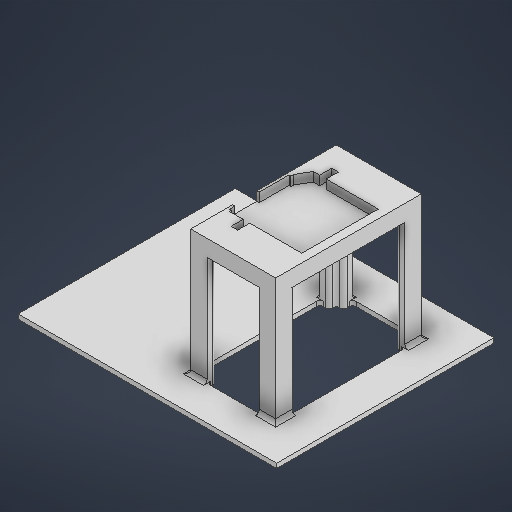
# Autodesk Inventor part: OMG_20kg_servo_side_profile(0.4mm)
Saved by Autodesk Inventor 2026.1 (Build 301233020, 233B)
## iProperties
Created: 2026-02-21
Part Number: OMG_20kg_servo_side_profile(0.4mm)
Material: Generic
Document SubType Name: Modeling
Designer: Lars
Density: 1 g/cm^3
Appearance: Default
Author: Lars
Autodesk Inventor part; units mm, degrees
ref_plane "YZ Plane" through (0, 0, 0) normal (1, 0, 0) x (0, 1, 0)
ref_plane "XZ Plane" through (0, 0, 0) normal (0, 1, 0) x (-1, 0, 0)
ref_plane "XY Plane" through (0, 0, 0) normal (0, 0, 1) x (1, 0, 0)
sketch "Sketch1" plane through (0, 0, 0) normal (0, 1, 0) x (-1, 0, 0)
  line L0 (0, 0) -> (28.63, 0)
  line L1 (28.63, 0) -> (28.63, -41.25) construction
  line L2 (28.63, -41.25) -> (0, -41.25)
  line L3 (0, -41.25) -> (0, 0)
  line L4 (28.63, 6.675) -> (31.43, 6.675)
  line L5 (31.43, 6.675) -> (31.43, 0)
  line L6 (31.43, -47.925) -> (28.63, -47.925)
  line L7 (28.63, -47.925) -> (28.63, -41.25)
  line L8 (31.43, -20.625) -> (28.63, -20.625) construction
  line L9 (38.98, 0) -> (31.43, 0)
  line L10 (31.43, 0) -> (31.43, -41.25) construction
  line L11 (31.43, -41.25) -> (35.18, -41.25)
  line L12 (38.98, -41.25) -> (38.98, -34.5) construction
  line L13 (31.43, -41.25) -> (35.18, -41.25) construction
  line L14 (38.98, 0) -> (38.98, -1) construction
  line L15 (38.98, -34.5) -> (35.18, -41.25)
  line L16 (38.98, -34.5) -> (38.98, -33)
  line L17 (35.18, -41.25) -> (38.98, -41.25) construction
  line L18 (38.98, 0) -> (38.98, -1) construction
  line L19 (38.98, -1) -> (39.98, -1)
  line L20 (39.98, -1) -> (39.98, -4)
  line L21 (39.98, -33) -> (38.98, -33)
  line L22 (38.98, -33) -> (38.98, -1) construction
  line L23 (38.98, -1) -> (38.98, -33) construction
  line L24 (38.98, -33) -> (38.98, -34.5) construction
  line L25 (38.98, -1) -> (38.98, 0)
  line L26 (38.98, -33) -> (38.98, -1) construction
  line L27 (31.43, 0) -> (31.43, -41.25) construction
  line L28 (31.43, -41.25) -> (31.43, -47.925)
  line L29 (28.63, -41.25) -> (28.63, 0) construction
  line L30 (28.63, 0) -> (28.63, 6.675)
  line L31 (28.63, 0) -> (31.43, 0) construction
  line L32 (31.43, -41.25) -> (28.63, -41.25) construction
  line L33 (39.98, -1) -> (39.98, -4) construction
  line L34 (39.98, -4) -> (41.28, -4)
  line L35 (41.28, -4) -> (41.28, -16.6)
  line L36 (41.28, -16.6) -> (39.98, -16.6)
  line L37 (39.98, -16.6) -> (39.98, -4) construction
  line L38 (39.98, -4) -> (39.98, -16.6) construction
  line L39 (39.98, -16.6) -> (39.98, -33)
  line L40 (41.68, -17) -> (41.68, -3.6)
  line L41 (41.68, -3.6) -> (40.38, -3.6)
  line L42 (40.38, -3.6) -> (40.38, -0.6)
  line L43 (40.38, -0.6) -> (39.38, -0.6)
  line L44 (39.38, -0.6) -> (39.38, 0.4)
  line L45 (39.38, 0.4) -> (31.83, 0.4)
  line L46 (31.83, 0.4) -> (31.83, 7.075)
  line L47 (31.83, 7.075) -> (28.23, 7.075)
  line L48 (28.23, 7.075) -> (28.23, 0.4)
  line L49 (28.23, 0.4) -> (-0.4, 0.4)
  line L50 (-0.4, 0.4) -> (-0.4, -41.65)
  line L51 (-0.4, -41.65) -> (28.23, -41.65)
  line L52 (28.23, -41.65) -> (28.23, -48.325)
  line L53 (28.23, -48.325) -> (31.83, -48.325)
  line L54 (31.83, -48.325) -> (31.83, -41.65)
  line L55 (31.83, -41.65) -> (35.4138, -41.65)
  line L56 (35.4138, -41.65) -> (39.38, -34.6049)
  line L57 (39.38, -34.6049) -> (39.38, -33.4)
  line L58 (39.38, -33.4) -> (40.38, -33.4)
  line L59 (40.38, -33.4) -> (40.38, -17)
  line L60 (40.38, -17) -> (41.68, -17)
  line L61 (0, -20.625) -> (39.98, -20.625) construction
  line L62 (44.99, 9.375) -> (-5.01, 9.375)
  line L63 (-5.01, 9.375) -> (-5.01, -50.625)
  line L64 (-5.01, -50.625) -> (44.99, -50.625)
  line L65 (44.99, -50.625) -> (44.99, 9.375)
  line L66 (19.99, 9.375) -> (19.99, -50.625) construction
  point P0 (30.03, 6.675)
  point P1 (19.99, -20.625)
  dimension "d0" = 28.63
  dimension "d1" = 41.25
  dimension "d2" = 2.8
  dimension "d3" = 54.6
  dimension "d4" = 7.55
  dimension "d5" = 41.25
  dimension "d6" = 3.75
  dimension "d7" = 34.5
  dimension "d8" = 1
  dimension "d9" = 32
  dimension "d10" = 1
  dimension "d11" = 6.675
  dimension "d12" = 3
  dimension "d13" = 1.3
  dimension "d14" = 12.6
  dimension "d15" = 0.4
  dimension "d16" = 50
  dimension "d17" = 60
  constraints: 134 end point, 35 parallel, 17 perpendicular, 8 midpoint, 7 horizontal, 5 vertical, 1 point on line, 20 other
  measures "d0" distance of L1.end L2.end
  measures "d1" distance of L0.end L1.end
  measures "d2" distance of L6.start L6.end
  measures "d3" distance of L4.end L6.start
  measures "d4" distance of L12.start L10.end
  measures "d5" distance of L12.start L9.start
  measures "d6" distance of L10.end L11.end
  measures "d7" distance of L9.start L12.end
  measures "d8" distance of L9.start L14.end
  measures "d9" distance of L19.end L21.start
  measures "d10" distance of L21.start L16.end
  measures "d11" distance from line of point (30.03, 6.675) L31
  measures "d12" distance of L19.end L20.end
  measures "d13" distance of L35.end L36.end
  measures "d14" distance of L34.end L35.end
  measures "d15" distance between parallel lines of L35 L40
  measures "d16" distance of L64.end L63.end
  measures "d17" distance of L63.end L62.end
extrude "Extrusion1" add sketch "Sketch1" along normal blind 5 contours L65 L64 L63 L62
sketch "Sketch2" plane through (0, 5, 0) normal (0, 1, 0) x (1, 0, 0)
  line L0 (-44.99, 50.625) -> (-44.99, -9.375) projected
  line L1 (5.01, 50.625) -> (-44.99, 50.625) projected
  line L2 (-44.99, -9.375) -> (-41.68, -9.375)
  line L3 (-41.68, -9.375) -> (-41.68, 50.625)
  line L4 (-41.68, 50.625) -> (-44.99, 50.625)
  line L5 (-44.99, 50.625) -> (-44.99, -9.375)
  point P0 (0, 0)
  dimension "d20" = 3.31
  constraints: 8 end point, 2 parallel, 1 horizontal, 1 perpendicular, 1 point on line
  measures "d20" distance of L4.end L3.end
extrude "Extrusion2" cut sketch "Sketch2" against normal through all
sketch "Sketch3" plane through (0, 0, 0) normal (0, -1, 0) x (1, 0, 0)
  line L0 (5.01, 9.375) -> (5.01, -50.625) projected
  line L1 (-41.68, -17) -> (-41.68, -50.625) projected
  line L2 (5.01, 9.375) -> (-41.68, 9.375)
  line L3 (-41.68, 9.375) -> (-41.68, -50.625)
  line L4 (-41.68, -50.625) -> (5.01, -50.625)
  line L5 (5.01, -50.625) -> (5.01, 9.375)
  point P0 (0, 0)
  constraints: 8 end point, 2 parallel, 1 horizontal, 1 perpendicular
extrude "Extrusion3" add sketch "Sketch3" along normal blind 4
sketch "Sketch4" plane through (-41.68, 5, 9.375) normal (0, 0, 1) x (1, 0, 0)
  line L0 (0, 0) -> (0, -9) projected
  line L1 (46.69, -9) -> (46.69, 0) projected
  line L2 (0, 0) -> (46.69, 0)
  line L3 (46.69, 0) -> (46.69, -9)
  line L4 (46.69, -9) -> (0, -9)
  line L5 (0, -9) -> (0, 0)
  point P0 (41.68, -5)
  constraints: 8 end point, 2 parallel, 1 horizontal, 1 perpendicular
extrude "Extrusion4" add sketch "Sketch4" along normal blind 10
sketch "Sketch5" plane through (5.01, 5, -50.625) normal (0, 0, -1) x (-1, 0, 0)
  line L0 (0, 0) -> (46.69, 0) projected
  line L1 (46.69, 0) -> (46.69, -9) projected
  line L2 (0, 0) -> (46.69, 0)
  line L3 (46.69, 0) -> (46.69, -9)
  line L4 (46.69, -9) -> (0, -9)
  line L5 (0, -9) -> (0, 0)
  point P0 (5.01, -5)
  constraints: 8 end point, 2 parallel, 1 horizontal, 1 perpendicular
extrude "Extrusion5" add sketch "Sketch5" along normal blind 10
sketch "Sketch6" plane through (0, -4, 0) normal (0, -1, 0) x (1, 0, 0)
  line L0 (-41.68, 19.375) -> (5.01, 19.375) projected
  line L1 (5.01, 19.375) -> (0.01, 19.375)
  line L2 (0.01, 14.375) -> (0.01, 10.375)
  line L3 (0.01, 10.375) -> (5.01, 10.375)
  line L4 (5.01, 10.375) -> (5.01, 19.375)
  line L5 (5.01, 19.375) -> (-3.99, 19.375)
  line L6 (-3.99, 19.375) -> (-3.99, 14.375)
  line L7 (-3.99, 14.375) -> (0.01, 14.375)
  line L8 (5.01, 14.375) -> (5.01, 19.375)
  point P0 (0, 0)
  dimension "d29" = 5
  dimension "d30" = 9
  dimension "d31" = 9
  dimension "d32" = 5
  constraints: 16 end point, 4 parallel, 2 horizontal, 2 perpendicular
  measures "d29" distance of L3.end L2.end
  measures "d30" distance of L2.end L1.end
  measures "d31" distance of L8.start L6.end
  measures "d32" distance of L6.end L5.end
extrude "Extrusion6" add sketch "Sketch6" along normal blind 60
sketch "Sketch7" plane through (0, -4, 0) normal (0, -1, 0) x (1, 0, 0)
  line L0 (5.01, -60.625) -> (5.01, 19.375) projected
  line L1 (5.01, -60.625) -> (-3.99, -60.625)
  line L2 (-3.99, -60.625) -> (-3.99, -55.625)
  line L3 (-3.99, -55.625) -> (0.01, -55.625)
  line L4 (5.01, -55.625) -> (5.01, -60.625)
  line L5 (5.01, -60.625) -> (0.01, -60.625)
  line L6 (0.01, -55.625) -> (0.01, -51.625)
  line L7 (0.01, -51.625) -> (5.01, -51.625)
  line L8 (5.01, -51.625) -> (5.01, -60.625)
  line L9 (-41.68, -60.625) -> (-41.68, 19.375) projected
  line L10 (-41.68, -60.625) -> (-32.68, -60.625)
  line L11 (-32.68, -60.625) -> (-32.68, -55.625)
  line L12 (-32.68, -55.625) -> (-36.68, -55.625)
  line L13 (-41.68, -55.625) -> (-41.68, -60.625)
  line L14 (-41.68, -60.625) -> (-36.68, -60.625)
  line L15 (-36.68, -55.625) -> (-36.68, -51.625)
  line L16 (-36.68, -51.625) -> (-41.68, -51.625)
  line L17 (-41.68, -51.625) -> (-41.68, -60.625)
  line L18 (-41.68, 19.375) -> (-32.68, 19.375)
  line L19 (-32.68, 19.375) -> (-32.68, 14.375)
  line L20 (-32.68, 14.375) -> (-36.68, 14.375)
  line L21 (-41.68, 14.375) -> (-41.68, 19.375)
  line L22 (-41.68, 19.375) -> (-36.68, 19.375)
  line L23 (-36.68, 14.375) -> (-36.68, 10.375)
  line L24 (-36.68, 10.375) -> (-41.68, 10.375)
  line L25 (-41.68, 10.375) -> (-41.68, 19.375)
  point P0 (0, 0)
  dimension "d35" = 9
  dimension "d36" = 5
  dimension "d37" = 5
  dimension "d38" = 9
  dimension "d39" = 9
  dimension "d40" = 5
  dimension "d41" = 5
  dimension "d42" = 9
  dimension "d43" = 9
  dimension "d44" = 5
  dimension "d45" = 5
  dimension "d46" = 9
  constraints: 48 end point, 12 parallel, 6 horizontal, 6 perpendicular
  measures "d35" distance of L2.end L4.start
  measures "d36" distance of L1.end L2.end
  measures "d37" distance of L6.end L7.end
  measures "d38" distance of L5.end L6.end
  measures "d39" distance of L13.start L11.end
  measures "d40" distance of L11.end L10.end
  measures "d41" distance of L16.end L15.end
  measures "d42" distance of L15.end L14.end
  measures "d43" distance of L19.end L21.start
  measures "d44" distance of L18.end L19.end
  measures "d45" distance of L23.end L24.end
  measures "d46" distance of L22.end L23.end
extrude "Extrusion7" add sketch "Sketch7" along normal blind 60
sketch "Sketch8" plane through (0, -64, 0) normal (0, -1, 0) x (1, 0, 0)
  line L0 (24.4558, -81.1334) -> (-117.6901, -81.1334)
  line L1 (-117.6901, -81.1334) -> (-117.6901, 38.2506)
  line L2 (-117.6901, 38.2506) -> (24.4558, 38.2506)
  line L3 (24.4558, 38.2506) -> (24.4558, -81.1334)
  point P0 (0, 0)
  constraints: 8 end point, 2 parallel, 1 horizontal, 1 perpendicular
extrude "Extrusion8" add sketch "Sketch8" along normal blind 2.5
sketch "Sketch9" plane through (0, -64, 0) normal (0, 1, 0) x (1, 0, 0)
  line L0 (-36.68, -10.375) -> (-36.68, -14.375) projected
  line L1 (0.01, 51.625) -> (0.01, 55.625) projected
  line L2 (-36.68, -14.375) -> (0.01, -14.375)
  line L3 (0.01, -14.375) -> (0.01, 55.625)
  line L4 (0.01, 55.625) -> (-36.68, 55.625)
  line L5 (-36.68, 55.625) -> (-36.68, -14.375)
  line L6 (-3.99, -19.375) -> (-32.68, -19.375)
  line L7 (-41.68, -10.375) -> (-41.68, 51.625)
  line L8 (-3.99, 60.625) -> (5.01, 60.625) projected
  line L9 (-32.68, 60.625) -> (-3.99, 60.625)
  line L10 (5.01, 51.5309) -> (5.01, -10.375)
  point P0 (0, 0)
  constraints: 16 end point, 2 horizontal, 2 parallel, 1 perpendicular, 1 vertical
extrude "Extrusion9" cut sketch "Sketch9" against normal blind 2.5
sketch "Sketch10" plane through (0, -64, 0) normal (0, 1, 0) x (1, 0, 0)
  line L0 (0.01, -10.375) -> (5.01, -10.375) projected
  line L1 (5.01, 51.625) -> (0.01, 51.625) projected
  line L2 (0.01, -10.375) -> (5.01, -10.375)
  line L3 (5.01, -10.375) -> (5.01, 51.625)
  line L4 (5.01, 51.625) -> (0.01, 51.625)
  line L5 (0.01, 51.625) -> (0.01, -10.375)
  line L6 (-3.99, 55.625) -> (-3.99, 60.625) projected
  line L7 (-32.68, 60.625) -> (-32.68, 55.625) projected
  line L8 (-3.99, 60.625) -> (-32.68, 60.625)
  line L9 (-32.68, 60.625) -> (-32.68, 55.625)
  line L10 (-32.68, 55.625) -> (-3.99, 55.625)
  line L11 (-3.99, 55.625) -> (-3.99, 60.625)
  line L12 (-36.68, 55.625) -> (-36.68, -14.375) projected
  line L13 (-36.68, 51.625) -> (-41.6778, 51.625)
  line L14 (-41.6778, 51.625) -> (-41.6778, -10.375)
  line L15 (-41.6778, -10.375) -> (-36.68, -10.375)
  line L16 (-36.68, -10.375) -> (-36.68, 51.625)
  line L17 (-3.99, -14.375) -> (-32.68, -14.375) projected
  line L18 (-32.68, -14.375) -> (-3.99, -14.375)
  line L19 (-3.99, -14.375) -> (-3.99, -19.375)
  line L20 (-3.99, -19.375) -> (-32.68, -19.375)
  line L21 (-32.68, -19.375) -> (-32.68, -14.375)
  point P0 (0, 0)
  constraints: 32 end point, 8 parallel, 4 horizontal, 4 perpendicular, 3 point on line
extrude "Extrusion10" cut sketch "Sketch10" against normal blind 2.5
fillet "Fillet1" radius 2 5 edges at (-3.99, -65.25, -60.625) (0.01, -35.25, -55.625) (0.01, -35.25, -51.625) (-3.99, -35.25, -55.625) (5.01, -65.25, -51.625)
fillet "Fillet2" radius 2 10 edges at (5.01, -65.25, 10.375) (0.01, -35.25, 10.375) (0.01, -35.25, 14.375) (-3.99, -35.25, 14.375) (-3.99, -65.25, 19.375) (-32.68, -65.25, 19.375) (-32.68, -35.25, 14.375) (-36.68, -35.25, 14.375) (-36.68, -35.25, 10.375) (-41.6778, -65.25, 10.375)
fillet "Fillet3" radius 2 5 edges at (-36.68, -35.25, -51.625) (-36.68, -35.25, -55.625) (-32.68, -35.25, -55.625) (-32.68, -65.25, -60.625) (-41.6778, -65.25, -51.625)
fillet "Fillet4" radius 2 8 edges at (-41.68, -64, -56.125) (-37.18, -64, -60.625) (-41.68, -64, 14.875) (-37.18, -64, 19.375) (0.51, -64, 19.375) (5.01, -64, 14.875) (5.01, -64, -56.125) (0.51, -64, -60.625)
equation "\"d5\" = d1"
body "Solid1"
